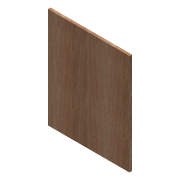
# Autodesk Inventor part: BellyPan for Drive in a Day
Saved by Autodesk Inventor 2013 (Build 170138000, 138)
## iProperties
Created: 2013-12-22
Part Number: BellyPan for Drive in a Day
Material: Wood (Birch)
Document SubType Name: Modeling
Designer: Nemo
Mass: 2345.07 g
Surface Area: 6495.63 cm^2
Volume: 3936.68 cm^3
Density: 0.595697 g/cm^3
Author: Nemo
Autodesk Inventor part; units mm, degrees
ref_plane "YZ Plane" through (0, 0, 0) normal (1, 0, 0) x (0, 1, 0)
ref_plane "XZ Plane" through (0, 0, 0) normal (0, 1, 0) x (-1, 0, 0)
ref_plane "XY Plane" through (0, 0, 0) normal (0, 0, 1) x (1, 0, 0)
sketch "Sketch1" plane through (0, 0, 0) normal (0, 0, 1) x (1, 0, 0)
  line L0 (-205.105, 273.05) -> (205.105, 273.05)
  line L1 (205.105, 273.05) -> (205.105, -273.05)
  line L2 (205.105, -273.05) -> (-205.105, -273.05)
  line L3 (-205.105, -273.05) -> (-205.105, 273.05)
  point P0 (0, 0)
  point P1 (-205.105, 0)
  point P2 (0, 273.05)
  dimension "d0" = 410.21
  dimension "d2" = 546.1
  constraints: 8 end point, 2 midpoint, 2 parallel, 1 horizontal, 1 horizontal alignment, 1 perpendicular, 1 vertical alignment
  measures "d0" distance of L0.start L0.end
  measures "d2" distance of L2.end L0.start
extrude "Extrusion1" add sketch "Sketch1" along normal blind 12.7
body "Solid1"
